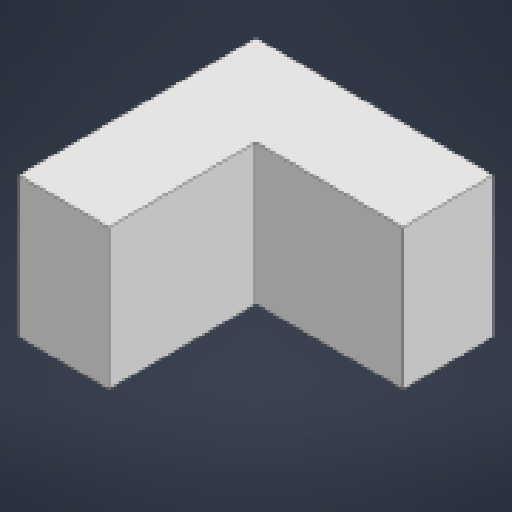
# Autodesk Inventor part: Pensile angolo
Saved by Autodesk Inventor 2024.2 (Build 282272000, 272)
## iProperties
Created: 2025-08-13
Part Number: Pensile angolo
Material: Generic
Document SubType Name: Modeling
Designer: Luca
Density: 1 g/cm^3
Appearance: Default
Author: Luca
Autodesk Inventor part; units mm, degrees
ref_plane "YZ Plane" through (0, 0, 0) normal (1, 0, 0) x (0, 1, 0)
ref_plane "XZ Plane" through (0, 0, 0) normal (0, 1, 0) x (-1, 0, 0)
ref_plane "XY Plane" through (0, 0, 0) normal (0, 0, 1) x (1, 0, 0)
sketch "Sketch1" plane through (0, 0, 0) normal (0, 1, 0) x (1, 0, 0)
  line L0 (0, 0) -> (0, -1050)
  line L1 (0, -1050) -> (400, -1050)
  line L2 (400, -1050) -> (400, -400)
  line L3 (0, 0) -> (1050, 0)
  line L4 (1050, 0) -> (1050, -400)
  line L5 (1050, -400) -> (400, -400)
  dimension "d1" = 1050
  dimension "d33" = 400
  constraints: 12 end point, 6 perpendicular, 1 coincident, 1 horizontal, 1 parallel
  measures "d1" distance of L0.start L0.end
  measures "d33" distance of L0.end L1.end
extrude "Extrusion1" add sketch "Sketch1" along normal blind 620
body "Solid1"
